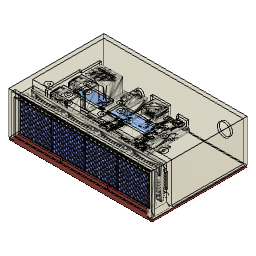
radio-v3 (Autodesk Fusion 360 design; units mm, degrees)
part number: 2025-08-03-13-42-16-987
part number: 2025-08-03-13-45-02-698
part number: 2025-08-07-17-49-59-308
part number: 2025-08-08-09-43-12-453
part number: 2025-08-09-19-33-53-891
Autodesk Fusion 360 part; units mm, degrees
other "Base Mesh Feature1" in component "Raspberry PI"
other "Modify1" in component "Raspberry PI"
other "Base Mesh Feature1'" in component "MAX"
sketch "Vrchni strana" plane through (0, 0, 0) normal (0, 0, 1) x (1, 0, 0) in component "vrsek"
  line L0 (0, 0) -> (142, 0)
  line L1 (142, 0) -> (142, 90)
  line L2 (142, 90) -> (0, 90)
  line L3 (0, 90) -> (0, 0)
  line L4 (0, 0) -> (142, 0)
  line L5 (142, 0) -> (142, 0.4)
  line L6 (142, 0.4) -> (0, 0.4)
  line L7 (0, 0.4) -> (0, 0)
  line L8 (0, 0) -> (2, 0)
  line L9 (2, 0) -> (2, 90)
  line L10 (2, 90) -> (0, 90)
  line L11 (0, 90) -> (0, 0)
  line L12 (0, 88) -> (0, 90)
  line L13 (35, 38) -> (61.5, 38)
  line L14 (61.5, 38) -> (61.5, 25)
  line L15 (61.5, 25) -> (35, 25)
  line L16 (35, 25) -> (35, 38)
  line L17 (68, 38) -> (107, 38)
  line L18 (107, 38) -> (107, 25)
  line L19 (107, 25) -> (68, 25)
  line L20 (68, 25) -> (68, 38)
  line L21 (142, 15.4) -> (0, 15.4)
  line L22 (0, 15.4) -> (0, 0.4)
  line L23 (142, 0) -> (140, 0)
  line L24 (140, 0) -> (140, 90)
  line L25 (140, 90) -> (142, 90)
  line L26 (142, 90) -> (142, 0)
  line L27 (142, 90) -> (0, 90)
  line L28 (0, 90) -> (0, 88)
  line L29 (0, 88) -> (142, 88)
  line L30 (142, 88) -> (142, 90)
  line L31 (0, 0) -> (5, 0)
  line L32 (5, 0) -> (5, 15.4)
  line L33 (5, 15.4) -> (0, 15.4)
  line L34 (0, 15.4) -> (0, 0)
  line L35 (142, 0) -> (137, 0)
  line L36 (137, 0) -> (137, 15.4)
  line L37 (137, 15.4) -> (142, 15.4)
  line L38 (142, 15.4) -> (142, 0)
  circle A0 centre (109, 22) radius 3
  circle A1 centre (109, 41) radius 3
  circle A2 centre (33, 41) radius 3
  circle A3 centre (33, 22) radius 3
  circle A4 centre (14, 21.4) radius 3.5
  circle A5 centre (128, 21.4) radius 3.5
  line L39 (0, 15.4) -> (142, 15.4)
  line L40 (142, 15.4) -> (142, 17.4)
  line L41 (142, 17.4) -> (0, 17.4)
  line L42 (0, 17.4) -> (0, 15.4)
  circle A6 centre (33, 22) radius 1.375
  circle A7 centre (33, 41) radius 1.375
  circle A8 centre (109, 41) radius 1.375
  circle A9 centre (109, 22) radius 1.375
  circle A10 centre (14, 21.4) radius 1.5
  circle A11 centre (128, 21.4) radius 1.5
  circle A12 centre (66, 41) radius 3
  circle A13 centre (66, 41) radius 1.375
  circle A14 centre (66, 22) radius 3
  circle A15 centre (66, 22) radius 1.375
  line L43 (0, 0) -> (142, 0)
  line L44 (142, 0) -> (142, -3.2)
  line L45 (142, -3.2) -> (0, -3.2)
  line L46 (0, -3.2) -> (0, 0)
  line L47 (0, -3.2) -> (142, -3.2)
  line L48 (142, -3.2) -> (142, -4.2)
  line L49 (142, -4.2) -> (0, -4.2)
  line L50 (0, -4.2) -> (0, -3.2)
  line L51 (2, 0) -> (2, -4.2)
  line L52 (140, 0) -> (140, -4.2)
  line L53 (137, -3.2) -> (137, -4.2)
  line L54 (5, -3.2) -> (5, -4.2)
  dimension "d1" = 142
  dimension "d2" = 90
  dimension "d3" = 0.4
  dimension "d4" = 2
  dimension "d5" = 2
  dimension "d7" = 26.5
  dimension "d8" = 13
  dimension "d9" = 35
  dimension "d10" = 39
  dimension "d13" = 6.5
  dimension "d14" = 15
  dimension "d16" = 25
  dimension "d17" = 2
  dimension "d18" = 2
  dimension "d19" = 5
  dimension "d20" = 5
  dimension "d21" = 6
  dimension "d22" = 2
  dimension "d23" = 3
  dimension "d24" = 6
  dimension "d25" = 19
  dimension "d26" = 6
  dimension "d27" = 6
  dimension "d28" = 76
  dimension "d29" = 7
  dimension "d30" = 14
  dimension "d31" = 6
  dimension "d32" = 7
  dimension "d33" = 14
  dimension "d36" = 2
  dimension "d41" = 2.75
  dimension "d42" = 2.75
  dimension "d43" = 2.75
  dimension "d44" = 2.75
  dimension "d45" = 3
  dimension "d46" = 3
  dimension "d69" = 6
  dimension "d70" = 2.75
  dimension "d71" = 33
  dimension "d72" = 6
  dimension "d73" = 2.75
  dimension "d343" = 3.2
  dimension "d344" = 1
  constraint horizontal L0
  constraint vertical L1
  constraint vertical L3
  constraint coincident L0.start L3.end
  constraint horizontal L4
  constraint vertical L5
  constraint horizontal L6
  constraint vertical L7
  constraint horizontal L8
  constraint vertical L9
  constraint horizontal L10
  constraint vertical L11
  constraint vertical L12
  constraint horizontal L13
  constraint vertical L14
  constraint horizontal L15
  constraint vertical L16
  constraint horizontal L17
  constraint vertical L18
  constraint horizontal L19
  constraint vertical L20
  constraint horizontal L14.end L19.end
  constraint horizontal L13.end L17.start
  constraint horizontal L21
  constraint vertical L22
  constraint perpendicular L1 L2
  constraint horizontal L23
  constraint vertical L24
  constraint horizontal L25
  constraint vertical L26
  constraint horizontal L1.end L24.end
  constraint horizontal L27
  constraint vertical L28
  constraint horizontal L29
  constraint vertical L30
  constraint horizontal L31
  constraint vertical L32
  constraint horizontal L33
  constraint vertical L34
  constraint horizontal L35
  constraint vertical L36
  constraint horizontal L37
  constraint vertical L38
  constraint vertical A0.centre A1.centre
  constraint horizontal A1.centre A2.centre
  constraint vertical A2.centre A3.centre
  constraint horizontal A0.centre A3.centre
  constraint horizontal A4.centre A5.centre
  constraint horizontal L39
  constraint vertical L40
  constraint horizontal L41
  constraint vertical L42
  constraint coincident L26 L40.end
  constraint vertical L0.end L21.start
  constraint horizontal L36.end L21.start
  constraint concentric A3 A6
  constraint concentric A2 A7
  constraint concentric A1 A8
  constraint concentric A0 A9
  constraint concentric A4 A10
  constraint concentric A5 A11
  constraint concentric A12 A13
  constraint horizontal A1.centre A12.centre
  constraint concentric A14 A15
  constraint vertical A12.centre A14.centre
  constraint horizontal A0.centre A14.centre
  constraint horizontal L21.end L32.end
  constraint vertical L12.start L2.end
  constraint horizontal L2.end L9.end
  constraint coincident L1.end L2.start
  constraint horizontal L43
  constraint vertical L44
  constraint horizontal L45
  constraint vertical L46
  constraint vertical L0.end L44.end
  constraint horizontal L47
  constraint vertical L48
  constraint horizontal L49
  constraint vertical L50
  constraint vertical L0.end L48.end
  constraint coincident L49 L51.end
  constraint perpendicular L49 L51
  constraint coincident L49 L52.end
  constraint perpendicular L49 L52
  constraint coincident L47 L53.start
  constraint coincident L49 L53.end
  constraint perpendicular L49 L53
  constraint vertical L35.end L53.start
  constraint coincident L47 L54.start
  constraint coincident L49 L54.end
  constraint perpendicular L49 L54
  constraint vertical L31.end L54.end
  measures "d1" distance of L0.start L0.end
  measures "d2" distance of L0.start L2.end
  measures "d3" distance of L0.start L6.end
  measures "d4" distance of L0.start L8.end
  measures "d5" distance of L2.end L12.start
  measures "d7" distance of L13.start L13.end
  measures "d8" distance of L13.start L15.end
  measures "d9" distance of L11 L15.end
  measures "d10" distance of L17.start L17.end
  measures "d13" distance of L14.end L19.end
  measures "d14" distance of L6.end L21.end
  measures "d16" vertical distance of L0.start L15.end
  measures "d17" distance of L0.end L23.end
  measures "d18" distance of L1.end L29.end
  measures "d19" distance of L0.start L31.end
  measures "d20" distance of L0.end L35.end
  measures "d21" diameter of A0
  measures "d22" horizontal distance of L18.end A0.centre
  measures "d23" vertical distance of L18.end A0.centre
  measures "d24" diameter of A1
  measures "d25" distance of A0.centre A1.centre
  measures "d26" diameter of A2
  measures "d27" diameter of A3
  measures "d28" distance of A1.centre A2.centre
  measures "d29" diameter of A4
  measures "d30" distance of L3 A4.centre
  measures "d31" distance of L21 A4.centre
  measures "d32" diameter of A5
  measures "d33" distance of L26 A5.centre
  measures "d36" distance of L21.start L40.end
  measures "d41" diameter of A6
  measures "d42" diameter of A7
  measures "d43" diameter of A8
  measures "d44" diameter of A9
  measures "d45" diameter of A10
  measures "d46" diameter of A11
  measures "d69" diameter of A12
  measures "d70" diameter of A13
  measures "d71" distance of A2.centre A12.centre
  measures "d72" diameter of A14
  measures "d73" diameter of A15
  measures "d343" vertical distance of L0.start L44.end
  measures "d344" distance of L45.end L49.end
extrude "Extrude9" add sketch "Vrchni strana" against normal blind 40 contours L0 L3 L4 L6 L7 L8 L9 L11 L31 L34 L43 | L0 L4 L8 L31 L43 L45 L46 L47 L51 | L0 L4 L6 L9 L31 L32 L43 | L3 L6 L9 L11 L21 L22 L33 L34 L39 | L45 L47 L49 L50 L51 | L6 L9 L21 L32 L33 L39 | L45 L47 L49 L51 L54 | L3 L9 L11 L21 L33 L39 L41 L42 | L0 L4 L6 L24 L35 L36 L43 | L9 L21 L24 L33 L37 L39 L41 | L3 L9 L11 L29 L41 | L0 L1 L4 L5 L6 L23 L24 L26 L35 L38 L43 | L0 L4 L23 L35 L43 L44 L45 L47 L52 | L6 L21 L24 L36 L37 L39 | L45 L47 L49 L52 L53 | L2 L3 L9 L10 L11 L12 L27 L28 L29 | L1 L6 L21 L24 L26 L37 L38 L39 | L45 L47 L48 L49 L52 | L2 L9 L24 L27 L29 | L1 L21 L24 L26 L37 L39 L40 L41 | L1 L24 L26 L29 L41 | L1 L2 L24 L25 L26 L27 L29 L30 makes body 1 in component "vrsek"
extrude "Extrude19" add sketch "Vrchni strana" against normal blind 3 contours L0 L4 L6 L32 L36 L43 | L6 L21 L32 L36 L39 bodies 1 in component "vrsek"
extrude "Extrude12" add sketch "Vrchni strana" 1 faces at (48, 11.6, 0) along normal blind 2 contours L0 L3 L4 L6 L7 L8 L9 L11 L31 L34 L43 | L0 L4 L8 L31 L43 L45 L46 L47 L51 | L0 L4 L6 L9 L31 L32 L43 | L0 L4 L31 L35 L43 L45 L47 L51 L52 | L3 L6 L9 L11 L21 L22 L33 L34 L39 | L45 L47 L49 L50 L51 | L0 L4 L6 L32 L36 L43 | L6 L9 L21 L32 L33 L39 | L45 L47 L49 L51 L54 | L3 L9 L11 L21 L33 L39 L41 L42 | L0 L4 L6 L24 L35 L36 L43 | L6 L21 L32 L36 L39 | L9 L21 L24 L33 L37 L39 L41 | L45 L47 L49 L53 L54 | L3 L9 L11 L29 L41 | L0 L1 L4 L5 L6 L23 L24 L26 L35 L38 L43 | L0 L4 L23 L35 L43 L44 L45 L47 L52 | L6 L21 L24 L36 L37 L39 | L9 L24 L29 L41 | L45 L47 L49 L52 L53 | L2 L3 L9 L10 L11 L12 L27 L28 L29 | L1 L6 L21 L24 L26 L37 L38 L39 | L45 L47 L48 L49 L52 | L2 L9 L24 L27 L29 | L1 L21 L24 L26 L37 L39 L40 L41 | L1 L24 L26 L29 L41 | L1 L2 L24 L25 L26 L27 L29 L30 | A0 | A1 | A2 | A3 | A4 | A5 | A6 | A7 | A8 | A9 | A10 | A11 | A12 | A13 | A14 | A15 on bodies 1 bodies 1 in component "vrsek"
extrude "Extrude20" add sketch "Vrchni strana" against normal blind 3 contours L45 L47 L49 L53 L54 bodies 1 in component "vrsek"
extrude "Extrude13" add sketch "Vrchni strana" against normal blind 7 contours A0 | A1 | A2 | A3 | A12 | A14 bodies 1 in component "vrsek"
extrude "Extrude14" add sketch "Vrchni strana" against normal blind 38 contours A4 | A5 bodies 1 in component "vrsek"
ref_plane "WorkPlane7" through (71, 42.9, -40) normal (0, 0, 1) x (1, 0, 0)
sketch "prostredni rovnina podlahy" plane through (0, 0, -40) normal (0, 0, 1) x (1, 0, 0) in component "spodek"
  line L0 (0, 0) -> (142, 0)
  line L1 (142, 0) -> (142, 90)
  line L2 (142, 90) -> (0, 90)
  line L3 (0, 90) -> (0, 0)
  line L4 (0, 88) -> (142, 88)
  line L5 (2, 0) -> (2, 90)
  line L6 (142, 17.4) -> (0, 17.4)
  line L7 (0, 15.4) -> (142, 15.4)
  line L8 (140, 0) -> (140, 90)
  line L9 (2, 88) -> (140, 88)
  line L10 (140, 88) -> (140, 17.4)
  line L11 (140, 17.4) -> (2, 17.4)
  line L12 (2, 17.4) -> (2, 88)
  line L13 (2, 15.4) -> (140, 15.4)
  line L14 (140, 15.4) -> (140, 0)
  line L15 (140, 0) -> (2, 0)
  line L16 (2, 0) -> (2, 15.4)
  line L17 (142, 0.4) -> (0, 0.4)
  line L18 (0, 0.4) -> (142, 0.4)
  circle A0 centre (128, 21.4) radius 3.5
  circle A1 centre (128, 21.4) radius 1.5
  circle A2 centre (14, 21.4) radius 3.5
  circle A3 centre (14, 21.4) radius 1.5
  circle A4 centre (86, 84) radius 3
  circle A5 centre (86, 84) radius 1.375
  circle A6 centre (28, 84) radius 3
  circle A7 centre (28, 84) radius 1.375
  circle A8 centre (86, 35) radius 3
  circle A9 centre (86, 35) radius 1.375
  circle A10 centre (28, 35) radius 3
  circle A11 centre (28, 35) radius 1.375
  line L19 (0, 0) -> (0, -3.2)
  line L20 (0, -3.2) -> (0, -4.2)
  line L21 (0, -4.2) -> (2, -4.2)
  line L22 (2, -4.2) -> (137, -4.2)
  line L23 (137, -4.2) -> (140, -4.2)
  line L24 (140, -4.2) -> (142, -4.2)
  line L25 (142, -4.2) -> (142, 0)
  line L26 (140, 0) -> (140, -3.2)
  line L27 (140, -3.2) -> (137, -3.2)
  line L28 (137, -3.2) -> (2, -3.2)
  line L29 (2, -3.2) -> (2, 0)
  line L30 (2, -3.2) -> (2, -4.2)
  line L31 (137, -3.2) -> (137, -4.2)
  line L32 (5, -3.2) -> (5, -4.2)
  line L33 (95, 0.4) -> (95, 15.4)
  line L34 (93.5, 15.4) -> (93.5, 0.4)
  line L35 (48.5, 15.4) -> (47, 15.4)
  line L36 (47, 15.4) -> (47, 0)
  line L37 (47, 0) -> (48.5, 0)
  line L38 (48.5, 0) -> (48.5, 15.4)
  line L39 (93.5, 0.4) -> (95, 0.4)
  line L40 (95, 0.4) -> (95, 0)
  line L41 (95, 0) -> (93.5, 0)
  line L42 (93.5, 0) -> (93.5, 0.4)
  point P0 (142, 90)
  point P1 (14, 21.4)
  point P2 (128, 21.4)
  point P3 (0, -4.2)
  point P4 (0, -3.2)
  point P5 (2, -4.2)
  point P6 (5, -4.2)
  point P7 (137, -3.2)
  point P8 (140, -4.2)
  point P9 (137, -4.2)
  point P10 (142, -4.2)
  point P11 (142, -3.2)
  point P12 (5, -3.2)
  dimension "d186" = 7
  dimension "d187" = 3
  dimension "d188" = 7
  dimension "d189" = 3
  dimension "d222" = 6
  dimension "d223" = 2.75
  dimension "d226" = 6
  dimension "d227" = 2.75
  dimension "d229" = 6
  dimension "d230" = 2.75
  dimension "d231" = 55
  dimension "d232" = 6
  dimension "d233" = 2.75
  dimension "d234" = 6
  dimension "d235" = 28
  dimension "d236" = 86
  dimension "d359" = 1.5
  dimension "d360" = 45
  dimension "d361" = 1.5
  dimension "d362" = 45
  dimension "d363" = 45
  constraint horizontal L0
  constraint vertical L1
  constraint horizontal L2
  constraint vertical L3
  constraint coincident L0.start L3.end
  constraint coincident P0 L1.end
  constraint horizontal L9
  constraint vertical L10
  constraint horizontal L11
  constraint vertical L12
  constraint coincident L8 L10.end
  constraint coincident L6 L10.end
  constraint coincident L5 L9.start
  constraint coincident L4 L9.start
  constraint horizontal L13
  constraint vertical L14
  constraint horizontal L15
  constraint vertical L16
  constraint coincident L8.start L14.end
  constraint coincident L5 L13.start
  constraint coincident L7 L13.start
  constraint coincident L17.end L18.start
  constraint coincident L17.start L18.end
  constraint coincident P2 A0.centre
  constraint concentric A0 A1
  constraint coincident P1 A2.centre
  constraint concentric A4 A5
  constraint concentric A6 A7
  constraint horizontal A4.centre A6.centre
  constraint concentric A8 A9
  constraint concentric A10 A11
  constraint vertical A6.centre A10.centre
  constraint vertical A4.centre A8.centre
  constraint horizontal A8.centre A10.centre
  constraint coincident P4 L19.end
  constraint coincident P3 L20.end
  constraint coincident P5 L21.end
  constraint coincident P9 L22.end
  constraint coincident P8 L23.end
  constraint coincident P10 L24.end
  constraint perpendicular L15 L26
  constraint coincident P7 L27.end
  constraint perpendicular L26 L27
  constraint perpendicular L20 L28
  constraint coincident L5.start L15.end
  constraint perpendicular L15 L29
  constraint coincident P12 L32.start
  constraint coincident P6 L32.end
  constraint vertical L33
  constraint coincident L18 L33.start
  constraint coincident L13 L33.end
  constraint coincident L7 L34.start
  constraint coincident L18 L34.end
  constraint perpendicular L18 L34
  constraint horizontal L35
  constraint vertical L36
  constraint horizontal L37
  constraint vertical L38
  constraint coincident L7 L35.start
  constraint coincident L15 L37.end
  constraint horizontal L39
  constraint vertical L40
  constraint horizontal L41
  constraint vertical L42
  constraint coincident L0 L40.end
  constraint vertical L33.start L40.end
  measures "d186" diameter of A0
  measures "d187" diameter of A1
  measures "d188" diameter of A2
  measures "d189" diameter of A3
  measures "d222" diameter of A4
  measures "d223" diameter of A5
  measures "d226" diameter of A6
  measures "d227" diameter of A7
  measures "d229" diameter of A8
  measures "d230" diameter of A9
  measures "d231" vertical distance of P0 A8.centre
  measures "d232" diameter of A10
  measures "d233" diameter of A11
  measures "d234" vertical distance of P0 A4.centre
  measures "d235" horizontal distance of L2.end A6.centre
  measures "d236" horizontal distance of L2.end A4.centre
  measures "d359" distance of L33.end L34.start
  measures "d360" horizontal distance of L8.start L33.start
  measures "d361" distance of L35.start L35.end
  measures "d362" distance of L13.start L35.end
  measures "d363" distance of L34.start L35.start
extrude "Extrude14'" add sketch "prostredni rovnina podlahy" against normal blind 2 separate body contours L0 L3 L5 L16 L17 L18 | L0 L19 L20 L21 L29 L30 | L0 L5 L15 L16 L17 L18 L36 | L0 L15 L26 L27 L28 L29 L37 L41 | L3 L5 L7 L16 L17 L18 | L0 L15 L17 L18 L36 L37 L38 | L5 L7 L13 L16 L17 L18 L36 | L22 L28 L30 L32 | L3 L5 L6 L7 | L0 L15 L17 L18 L38 L42 | L7 L13 L17 L18 L35 L36 L38 | L5 L6 L7 L8 L11 L13 L35 | L22 L28 L31 L32 | L3 L4 L5 L6 L12 | L0 L15 L17 L18 L39 L40 L41 L42 | L7 L13 L17 L18 L34 L38 | L4 L5 L6 L8 L9 L10 L11 L12 | L0 L23 L24 L25 L26 L27 L31 | L2 L3 L4 L5 | L0 L8 L14 L15 L17 L18 L40 | L7 L13 L17 L18 L33 L34 L39 | L2 L4 L5 L8 L9 | L1 L4 L6 L8 L10 | L1 L6 L7 L8 | L0 L1 L8 L14 L17 L18 | L7 L8 L13 L14 L17 L18 L33 | L1 L2 L4 L8 | L1 L7 L8 L14 L17 L18 | A0 | A1 | A2 | A3 | A4 | A5 | A6 | A7 | A8 | A9 | A10 | A11 makes body 2 in component "spodek"
extrude "Extrude6" add sketch "prostredni rovnina podlahy" along normal blind 1 contours L4 L5 L6 L8 L9 L10 L11 L12 | A0 | A1 | A2 | A3 | A4 | A5 | A6 | A7 | A8 | A9 | A10 | A11 bodies 2 in component "spodek"
extrude "Extrude13'" add sketch "prostredni rovnina podlahy" along normal blind 3 contours L0 L5 L15 L16 L17 L18 L36 | L5 L7 L13 L16 L17 L18 L36 | L0 L15 L17 L18 L38 L42 | L7 L13 L17 L18 L34 L38 | L0 L8 L14 L15 L17 L18 L40 | L7 L8 L13 L14 L17 L18 L33 bodies 2 in component "spodek"
extrude "Extrude8" add sketch "prostredni rovnina podlahy" along normal blind 2 contours A0 | A1 | A2 | A3 bodies 2 in component "spodek"
extrude "Extrude15" add sketch "prostredni rovnina podlahy" along normal blind 3 contours L22 L28 L31 L32 bodies 2 in component "spodek"
thread "Thread3" "ISO Metric profile 3.0 M3x0.5 M3x0.5 6H" major diameter 3.086 minor diameter 2.529 pitch 0.5 angle 60 resizes the face on face at (109.171, 23.3643, -4.6667) on bodies 1 in component "vrsek"
thread "Thread4" "ISO Metric profile 3.0 M3x0.5 M3x0.5 6H" major diameter 3.086 minor diameter 2.529 pitch 0.5 angle 60 resizes the face on face at (109.171, 42.3643, -4.6667) on bodies 1 in component "vrsek"
thread "Thread5" "ISO Metric profile 3.0 M3x0.5 M3x0.5 6H" major diameter 3.086 minor diameter 2.529 pitch 0.5 angle 60 resizes the face on face at (65.829, 23.3643, -4.6667) on bodies 1 in component "vrsek"
thread "Thread6" "ISO Metric profile 3.0 M3x0.5 M3x0.5 6H" major diameter 3.086 minor diameter 2.529 pitch 0.5 angle 60 resizes the face on face at (66.171, 42.3643, -4.6667) on bodies 1 in component "vrsek"
thread "Thread7" "ISO Metric profile 3.0 M3x0.5 M3x0.5 6H" major diameter 3.086 minor diameter 2.529 pitch 0.5 angle 60 resizes the face on face at (34.3682, 21.8631, -4.6667) on bodies 1 in component "vrsek"
thread "Thread8" "ISO Metric profile 3.0 M3x0.5 M3x0.5 6H" major diameter 3.086 minor diameter 2.529 pitch 0.5 angle 60 resizes the face on face at (34.2921, 40.5297, -4.6667) on bodies 1 in component "vrsek"
thread "Thread9" "ISO Metric profile 3.0 M3x0.5 M3x0.5 6H" major diameter 3.086 minor diameter 2.529 pitch 0.5 angle 60 resizes the face on face at (12.5075, 21.2506, -25.3333) from (14, 21.4, -28) to (14, 21.4, -38) on bodies 1 in component "vrsek"
thread "Thread10" "ISO Metric profile 3.0 M3x0.5 M3x0.5 6H" major diameter 3.086 minor diameter 2.529 pitch 0.5 angle 60 resizes the face on face at (128.6843, 22.7348, -25.3333) from (128, 21.4, -28) to (128, 21.4, -38) on bodies 1 in component "vrsek"
extrude "Extrude9'" add sketch "prostredni rovnina podlahy" along normal blind 4 contours A4 | A5 | A6 | A7 | A8 | A9 | A10 | A11 bodies 2 in component "spodek"
sketch "vrtani distancnich sloupku rpistancnich" plane through (0, 0, -40) normal (0, 0, 1) x (1, 0, 0) in component "spodek"
  point P0 (28, 35)
  point P1 (28, 84)
  point P2 (86, 84)
  point P3 (86, 35)
ref_plane "WorkPlane3" through (0, 90, 0) normal (0, 1, 0) x (0, 0, 1)
sketch "zadni" plane through (0, 90, 0) normal (0, 1, 0) x (1, 0, 0) in component "vrsek"
  line L0 (48.5, 26) -> (66.5, 26)
  line L1 (66.5, 26) -> (66.5, 40)
  line L2 (66.5, 40) -> (48.5, 40)
  line L3 (48.5, 40) -> (48.5, 26)
  line L4 (74, 30) -> (84, 30)
  line L5 (84, 30) -> (84, 40)
  line L6 (84, 40) -> (74, 40)
  line L7 (74, 40) -> (74, 30)
  circle A0 centre (36, 31) radius 4
  line L8 (0, 40) -> (0, 0)
  circle A1 centre (121, 19) radius 6.5
  line L9 (142, -2) -> (142, 40)
  line L10 (142, 40) -> (0, 40)
  line L11 (0, 40) -> (0, -2)
  line L12 (0, -2) -> (142, -2)
  point P0 (142, -2)
  dimension "d256" = 8
  dimension "d257" = 36
  dimension "d258" = 18
  dimension "d259" = 10
  dimension "d260" = 7.5
  dimension "d261" = 12.5
  dimension "d262" = 10
  dimension "d263" = 9
  dimension "d264" = 14
  dimension "d269" = 13
  dimension "d270" = 21
  dimension "d271" = 21
  constraint horizontal L0
  constraint vertical L1
  constraint horizontal L2
  constraint vertical L3
  constraint horizontal L4
  constraint vertical L5
  constraint horizontal L6
  constraint vertical L7
  constraint horizontal L2.end L8.start
  constraint horizontal L6.end L8.start
  measures "d256" diameter of A0
  measures "d257" distance of A0.centre L8
  measures "d258" distance of L1.end L2.end
  measures "d259" distance of L5.end L6.end
  measures "d260" horizontal distance of L1.end L6.end
  measures "d261" horizontal distance of L2.end A0.centre
  measures "d262" distance of L4.end L5.end
  measures "d263" vertical distance of A0.centre L8.start
  measures "d264" distance of L0 L8.start
  measures "d269" diameter of A1
  measures "d270" vertical distance of A1.centre P0
  measures "d271" horizontal distance of A1.centre P0
extrude "Extrude16" cut sketch "zadni" against normal blind 2 contours L0 L1 L2 L3 L10 | L4 L5 L6 L7 L10 | A0 | A1 bodies 1 in component "vrsek"
extrude "Extrude11" [no effect] in component "spodek"
sketch "bocni" plane through (0, 0, 0) normal (1, 0, 0) x (0, 1, 0) in component "vrsek"
  line L0 (86, -19) -> (68, -19)
  line L1 (68, -19) -> (68, -40)
  line L2 (68, -40) -> (86, -40)
  line L3 (86, -40) -> (86, -19)
  line L4 (66, -40) -> (50, -40)
  line L5 (50, -40) -> (50, -17)
  line L6 (50, -17) -> (66, -17)
  line L7 (66, -17) -> (66, -40)
  line L8 (48, -40) -> (32, -40)
  line L9 (32, -40) -> (32, -17)
  line L10 (32, -17) -> (48, -17)
  line L11 (48, -17) -> (48, -40)
  line L12 (68, -19) -> (66, -19)
  line L13 (68, -40) -> (66, -40)
  line L14 (50, -40) -> (48, -40)
  line L15 (50, -17) -> (48, -17)
  point P0 (90, 2)
  point P1 (90, -40)
  dimension "d276" = 21
  dimension "d277" = 16
  dimension "d278" = 2
  dimension "d279" = 16
  dimension "d280" = 2
  dimension "d281" = 18
  dimension "d282" = 4
  dimension "d283" = 23
  constraint horizontal L0
  constraint vertical L1
  constraint horizontal L2
  constraint vertical L3
  constraint horizontal L4
  constraint vertical L5
  constraint horizontal L6
  constraint vertical L7
  constraint horizontal L8
  constraint vertical L9
  constraint horizontal L10
  constraint vertical L11
  constraint horizontal L5.end L10.end
  constraint horizontal L2.end P1
  constraint horizontal L4.start P1
  constraint horizontal L8.start P1
  constraint coincident L7 L12.end
  constraint perpendicular L7 L12
  measures "d276" distance of L0.start L2.end
  measures "d277" distance of L8.start L8.end
  measures "d278" distance of L4.end L8.start
  measures "d279" distance of L4.start L4.end
  measures "d280" horizontal distance of L1.end L4.start
  measures "d281" distance of L1.end L2.end
  measures "d282" horizontal distance of L2.end P0
  measures "d283" distance of L8.end L9.end
extrude "Extrude17" cut sketch "bocni" along normal blind 2 bodies 1 in component "vrsek"
other "MeshRepair1" in component "Raspberry PI"
hole "Hole3" at (86, 35, -40) at (28, 35, -40) at (28, 84, -40) at (86, 84, -40) direction (0, 0, 1) diameter 2.529 depth 5 tip angle 180 bodies 2 in component "spodek"
thread "Thread3'" "ISO Metric profile 3.0 M3x0.5 M3x0.5 6H" major diameter 3.086 minor diameter 2.529 pitch 0.5 angle 60 resizes the face on face at (86.2506, 85.2394, -38.6667) on face at (26.7453, 84.1572, -38.6667) on face at (26.7359, 35.0315, -38.6667) on face at (86.2506, 36.2394, -38.6667) on bodies 2 in component "spodek"
ref_plane "WorkPlane2" through (0, 90, 0) normal (0, 1, 0) x (0, 0, 1)
ref_plane "WorkPlane4" through (0, 15.2, 0) normal (0, 1, 0) x (0, 0, 1)
sketch "vnitrni" plane through (0, 15.2, 0) normal (0, 1, 0) x (1, 0, 0) in component "vrsek"
  line L0 (6, 12) -> (8.5, 12)
  line L1 (8.5, 12) -> (8.5, 27)
  line L2 (8.5, 27) -> (6, 27)
  line L3 (6, 27) -> (6, 12)
  circle A0 centre (9, 9) radius 1.5
  circle A1 centre (9, 30) radius 1.5
  line L4 (133, 12) -> (136, 12)
  line L5 (136, 12) -> (136, 27)
  line L6 (136, 27) -> (133, 27)
  line L7 (133, 27) -> (133, 12)
  circle A2 centre (133.5, 9) radius 1.5
  circle A3 centre (133.5, 30) radius 1.5
  point P0 (0, -2)
  point P1 (5, 40)
  point P2 (5, 3)
  point P3 (137, 40)
  point P4 (137, 3)
  dimension "d287" = 3
  dimension "d288" = 3
  dimension "d289" = 2.5
  dimension "d290" = 15
  dimension "d291" = 3
  dimension "d292" = 3
  dimension "d293" = 3
  dimension "d294" = 12
  dimension "d296" = 3
  dimension "d297" = 3
  dimension "d298" = 3
  dimension "d299" = 3
  dimension "d300" = 3
  dimension "d301" = 2.5
  dimension "d305" = 2
  constraint horizontal L0
  constraint vertical L1
  constraint horizontal L2
  constraint vertical L3
  constraint vertical A0.centre A1.centre
  constraint horizontal L4
  constraint vertical L5
  constraint horizontal L6
  constraint vertical L7
  constraint horizontal L2.end L6.end
  constraint horizontal L0.start L4.start
  constraint vertical A2.centre A3.centre
  measures "d287" diameter of A1
  measures "d288" diameter of A0
  measures "d289" distance of L1.end L2.end
  measures "d290" distance of L0.start L2.end
  measures "d291" vertical distance of L0.start A0.centre
  measures "d292" vertical distance of L2.end A1.centre
  measures "d293" horizontal distance of L2.end A1.centre
  measures "d294" vertical distance of origin L0.start
  measures "d296" distance of L5.end L6.end
  measures "d297" diameter of A2
  measures "d298" diameter of A3
  measures "d299" vertical distance of L4.start A2.centre
  measures "d300" vertical distance of L6.end A3.centre
  measures "d301" horizontal distance of L4.end A2.centre
  measures "d305" distance of P0 origin
extrude "Extrude18" cut sketch "vnitrni" along normal blind 2 bodies 1 in component "vrsek"
other "Modify1'" in component "MAX"
sketch "kraj pod dirky" plane through (0, 0, -42) normal (0, 0, 1) x (1, 0, 0) in component "spodek"
  line L0 (2, 0) -> (2, 90)
  line L1 (142, -4.2) -> (142, 90)
  line L2 (142, 90) -> (0, 90)
  line L3 (0, 90) -> (0, -4.2)
  line L4 (61.5, 25) -> (35, 25)
  line L5 (35, 25) -> (35, 38)
  line L6 (35, 38) -> (61.5, 38)
  line L7 (61.5, 38) -> (61.5, 25)
  line L8 (107, 25) -> (68, 25)
  line L9 (68, 25) -> (68, 38)
  line L10 (68, 38) -> (107, 38)
  line L11 (107, 38) -> (107, 25)
  line L12 (0, 90) -> (0, 0)
  line L13 (0, 88) -> (142, 88)
  line L14 (142, 90) -> (0, 90)
  line L15 (84, 90) -> (74, 90)
  line L16 (74, 90) -> (74, 88)
  line L17 (74, 88) -> (84, 88)
  line L18 (84, 88) -> (84, 90)
  line L19 (66.5, 90) -> (48.5, 90)
  line L20 (48.5, 90) -> (48.5, 88)
  line L21 (48.5, 88) -> (66.5, 88)
  line L22 (66.5, 88) -> (66.5, 90)
  line L23 (0, 86) -> (2, 86)
  line L24 (2, 86) -> (2, 68)
  line L25 (2, 68) -> (0, 68)
  line L26 (0, 68) -> (0, 86)
  line L27 (0, 66) -> (2, 66)
  line L28 (2, 66) -> (2, 50)
  line L29 (2, 50) -> (0, 50)
  line L30 (0, 50) -> (0, 66)
  line L31 (0, 48) -> (2, 48)
  line L32 (2, 48) -> (2, 32)
  line L33 (2, 32) -> (0, 32)
  line L34 (0, 32) -> (0, 48)
  line L35 (0, -4.2) -> (142, -4.2)
  line L36 (142, 90) -> (142, -4.2)
  line L37 (142, -4.2) -> (0, -4.2)
  line L38 (0, -4.2) -> (0, 90)
  line L39 (0, 90) -> (142, 90)
  point P0 (0, 48)
  point P1 (0, 50)
  point P2 (0, 32)
  point P3 (0, 66)
  point P4 (0, 68)
  point P5 (0, 86)
  point P6 (48.5, 90)
  point P7 (66.5, 90)
  point P8 (74, 90)
  point P9 (84, 90)
  point P10 (48.5, 90)
  point P11 (14, 21.4)
  point P12 (128, 21.4)
  constraint horizontal L15
  constraint vertical L16
  constraint horizontal L17
  constraint vertical L18
  constraint coincident L13 L16.end
  constraint coincident P9 L15.start
  constraint horizontal L19
  constraint vertical L20
  constraint horizontal L21
  constraint vertical L22
  constraint coincident L13 L20.end
  constraint coincident P7 L19.start
  constraint horizontal L23
  constraint vertical L24
  constraint horizontal L25
  constraint vertical L26
  constraint coincident L0 L24.end
  constraint coincident P5 L23.start
  constraint horizontal L27
  constraint vertical L28
  constraint horizontal L29
  constraint vertical L30
  constraint coincident L0 L28.end
  constraint coincident P3 L27.start
  constraint horizontal L31
  constraint vertical L32
  constraint horizontal L33
  constraint vertical L34
  constraint coincident L0 L32.end
  constraint coincident P0 L31.start
  constraint coincident P8 L15.end
  constraint vertical L20.end P10
  constraint horizontal P4 L24.end
  constraint horizontal P1 L28.end
  constraint horizontal P2 L32.end
extrude "Extrude12'" add sketch "kraj pod dirky" along normal blind 7 contours L0 L3 L12 L31 L32 L33 L34 L38 | L0 L3 L12 L29 L31 L38 | L0 L3 L12 L27 L28 L29 L30 L38 | L0 L3 L12 L25 L27 L38 | L0 L3 L12 L23 L24 L25 L26 L38 | L2 L13 L14 L15 L16 L17 L18 L39 | L2 L13 L14 L19 L20 L21 L22 L39 bodies 2 in component "spodek"
sketch "Sketch9" plane through (0, 0, -39) normal (0, 0, -1) x (1, 0, 0)
  line L0 (142, -90) -> (142, 0)
  line L1 (142, 0) -> (0, 0)
  line L2 (0, 0) -> (0, -90)
  line L3 (0, -90) -> (142, -90)
  line L4 (0, 3.6) -> (142, 3.6)
  line L5 (142, 3.6) -> (142, -90)
  line L6 (142, -90) -> (0, -90)
  line L7 (0, -90) -> (0, 3.6)
  line L8 (107, -25) -> (68, -25)
  line L9 (68, -25) -> (68, -38)
  line L10 (68, -38) -> (107, -38)
  line L11 (107, -38) -> (107, -25)
  line L12 (61.5, -25) -> (35, -25)
  line L13 (35, -25) -> (35, -38)
  line L14 (35, -38) -> (61.5, -38)
  line L15 (61.5, -38) -> (61.5, -25)
  circle A0 centre (86, -84) radius 3
  circle A1 centre (86, -35) radius 3
  circle A2 centre (28, -84) radius 3
  circle A3 centre (28, -35) radius 3
  circle A4 centre (128, -21.4) radius 3.5
  circle A5 centre (14, -21.4) radius 3.5
  line L16 (2, -17.4) -> (140, -17.4)
  line L17 (140, -17.4) -> (140, -88)
  line L18 (140, -88) -> (84, -88)
  line L19 (84, -88) -> (74, -88)
  line L20 (66.5, -88) -> (48.5, -88)
  line L21 (48.5, -88) -> (2, -88)
  line L22 (2, -88) -> (2, -86)
  line L23 (2, -86) -> (2, -32)
  line L24 (2, -32) -> (2, -17.4)
  line L25 (74, -88) -> (66.5, -88)
  point P0 (14, -21.4)
  point P1 (128, -21.4)
hole "Hole6" at (14, 21.4, -39) at (128, 21.4, -39) direction (0, 0, 1) diameter 3 depth 10 tip angle 180 countersink diameter 5 countersink angle 90 bodies 2 in component "spodek"
chamfer "Chamfer6" distance 3 angle 45 2 edges at (140, 7.7, -37) (2, 7.7, -37) on bodies 2 in component "spodek"
chamfer "Chamfer6" distance 1 angle 45 6 edges at (140, 52.7, -39) (2, 24.7, -39) (25.25, 88, -39) (70.25, 88, -39) (112, 88, -39) (2, 87, -39) on bodies 2 in component "spodek"
hole "Hole7" at (14, 21.4, -42) direction (0, 0, 1) diameter 3 depth 10 tip angle 118 countersink diameter 6 countersink angle 90 bodies 2 in component "spodek"
hole "Hole8" at (128, 21.4, -42) direction (0, 0, 1) diameter 3 depth 10 tip angle 118 countersink diameter 6 countersink angle 90 bodies 2 in component "spodek"
chamfer "Chamfer3" distance 3 angle 45 2 edges at (137, 7.7, -40) (5, 7.7, -40) on bodies 1 in component "vrsek"
chamfer "Chamfer3" distance 1 angle 45 6 edges at (140, 52.7, -40) (112, 88, -40) (70.25, 88, -40) (25.25, 88, -40) (2, 87, -40) (2, 24.7, -40) on bodies 1 in component "vrsek"
component "vrsek" placed x (1, 0, 0) y (0, 1, 0) z (0, 0, 1) at (0, 0, 0)
component "Raspberry PI" placed x (1, 0, 0) y (0, 1, 0) z (0, 0, 1) at (0, 0, 0)
component "MAX" placed x (1, 0, 0) y (0, 1, 0) z (0, 0, 1) at (0, 0, 0)
component "spodek" placed x (1, 0, 0) y (0, 1, 0) z (0, 0, 1) at (0, 0, 0)
